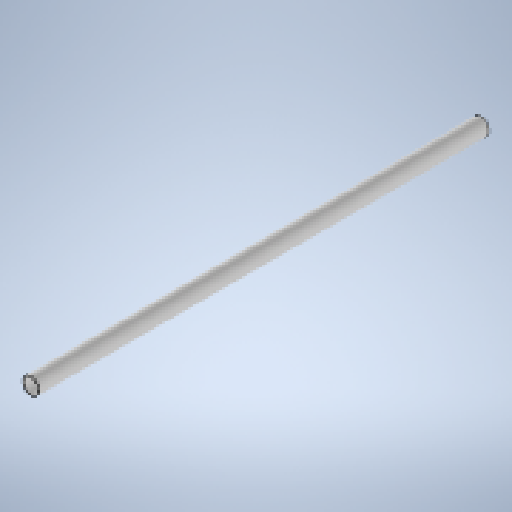
# Autodesk Inventor part: MSC 618 belly tube 18
Saved by Autodesk Inventor 2025 (Build 290162010, 162A)
## iProperties
Created: 2024-05-24
Part Number: MSC 618 belly tube 18
Material: Generic
Document SubType Name: Modeling
Designer: user
Stock Number: МОО 606 ракета труба 6
Density: 1 g/cm^3
Appearance: Default
Author: admin
Autodesk Inventor part; units mm, degrees
ref_plane "YZ Plane" through (0, 0, 0) normal (1, 0, 0) x (0, 1, 0)
ref_plane "XZ Plane" through (0, 0, 0) normal (0, 1, 0) x (-1, 0, 0)
ref_plane "XY Plane" through (0, 0, 0) normal (0, 0, 1) x (1, 0, 0)
sketch "Sketch1" plane through (0, 0, 0) normal (0, 0, 1) x (1, 0, 0)
  circle A0 centre (0, 0) radius 38.05
  circle A1 centre (0, 0) radius 35.05
  dimension "d0" = 76.1
  dimension "d1" = 3
  constraints: 2 centre point, 1 coincident
  measures "d0" diameter of A0
  measures "d1" radial gap between concentric circles of A0 A1
extrude "Extrusion1" add sketch "Sketch1" along normal blind 2050
body "Solid1"
